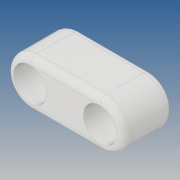
# Autodesk Inventor part: 链
Saved by Autodesk Inventor 2019.1 (Build 231200000, 200)
## iProperties
Company: 北京理工大学
Created: 2020-09-30
Part Number: 链
Material: ABS 塑料
Document SubType Name: Modeling
Designer: 谢庆红冰
Density: 1.06 g/cm^3
Appearance: 平滑 - 白色
Author: 谢庆红冰
Autodesk Inventor part; units mm, degrees
ref_plane "YZ Plane" through (0, 0, 0) normal (1, 0, 0) x (0, 1, 0)
ref_plane "XZ Plane" through (0, 0, 0) normal (0, 1, 0) x (-1, 0, 0)
ref_plane "XY Plane" through (0, 0, 0) normal (0, 0, 1) x (1, 0, 0)
sketch "草图1" plane through (0, 0, 0) normal (0, 0, 1) x (1, 0, 0)
  circle A0 centre (9, 0) radius 2.5 construction
  circle A1 centre (0, 0) radius 2.5 construction
  circle A2 centre (0, 0) radius 2.5
  circle A3 centre (0, 0) radius 3.5
  line L0 (10.5, 3.5) -> (0, 3.5)
  line L1 (0, -3.5) -> (10.5, -3.5)
  circle A4 centre (10.5, 0) radius 2.5 construction
  circle A5 centre (10.5, 0) radius 2.5
  circle A6 centre (10.5, 0) radius 3.5
  line L2 (0, 0) -> (9.7373, 0) construction
  point P0 (1, 4.5)
  point P1 (1, -2.5)
  dimension "d4" = 7
  dimension "d7" = 7
  dimension "d8" = 10.5
  dimension "d9" = 10.5
  constraints: 6 end point, 5 centre point, 4 coincident, 4 point on circle, 2 concentric, 2 horizontal, 1 parallel, 1 point on line, 1 tangent
  measures "d4" diameter of A3
  measures "d7" diameter of A6
  measures "d8" distance of L1.start L1.end
  measures "d9" distance of L0.start L0.end
extrude "拉伸1" add sketch "草图1" along normal mid plane 7.5
fillet "圆角1" radius 1 8 edges at (-3.5, 0, 3.75) (5.25, -3.5, 3.75) (14, 0, 3.75) (5.25, 3.5, 3.75) (14, 0, -3.75) (5.25, -3.5, -3.75) (-3.5, 0, -3.75) (5.25, 3.5, -3.75)
equation "\"d9\" = d8"
